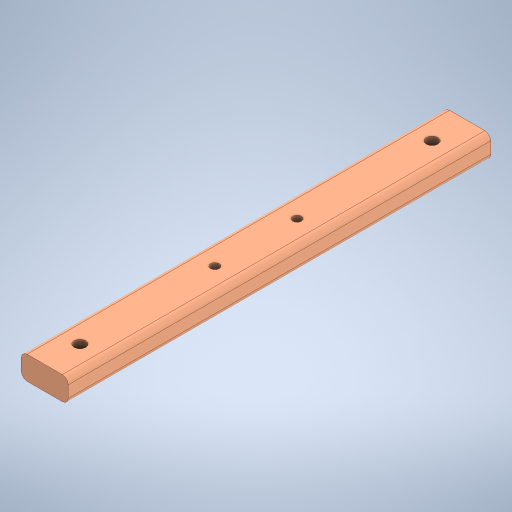
# Autodesk Inventor part: Wood-4
Saved by Autodesk Inventor 2024 (Build 280153000, 153)
## iProperties
Created: 2024-03-20
Part Number: Wood-4
Material: Generic
Document SubType Name: Modeling
Designer: Liz
Density: 1 g/cm^3
Appearance: Default
Author: Liz
Autodesk Inventor part; units mm, degrees
ref_plane "YZ Plane" through (0, 0, 0) normal (1, 0, 0) x (0, 1, 0)
ref_plane "XZ Plane" through (0, 0, 0) normal (0, 1, 0) x (-1, 0, 0)
ref_plane "XY Plane" through (0, 0, 0) normal (0, 0, 1) x (1, 0, 0)
sketch "Sketch1" plane through (0, 0, 0) normal (0, 0, 1) x (1, 0, 0)
  line L0 (-38.1, -25.4) -> (38.1, -25.4)
  line L1 (50.8, -12.7) -> (50.8, 12.7)
  line L2 (38.1, 25.4) -> (-38.1, 25.4)
  line L3 (-50.8, 12.7) -> (-50.8, -12.7)
  line L4 (-50.8, -25.4) -> (50.8, 25.4) construction
  line L5 (50.8, -25.4) -> (-50.8, 25.4) construction
  arc A0 (-38.1, 25.4) -> (-50.8, 12.7) centre (-38.1, 12.7) ccw
  arc A1 (-50.8, -12.7) -> (-38.1, -25.4) centre (-38.1, -12.7) ccw
  arc A2 (38.1, -25.4) -> (50.8, -12.7) centre (38.1, -12.7) ccw
  arc A3 (50.8, 12.7) -> (38.1, 25.4) centre (38.1, 12.7) ccw
  point P0 (0, 0)
  dimension "d0" = 50.8
  dimension "d1" = 101.6
  dimension "d2" = 12.7
  constraints: 12 end point, 8 point on circle, 8 point on line, 8 tangent, 4 centre point, 3 equal radius, 2 midpoint, 2 parallel, 1 horizontal, 1 perpendicular
  measures "d0" distance of L5.end L4.start
  measures "d1" distance of L4.end L5.end
  measures "d2" radius of A0
extrude "Extrusion1" add sketch "Sketch1" along normal blind 914.4
sketch "Sketch2" plane through (-38.1, 25.4, 0) normal (0, 1, 0) x (1, 0, 0)
  circle A0 centre (38.1, -838.2) radius 12.7
  circle A1 centre (38.1, -76.2) radius 12.7
  line L0 (76.2, 0) -> (0, 0) projected
  line L1 (-12.7, 0) -> (-12.7, -914.4) projected
  circle A2 centre (38.1, -546.1) radius 9.525
  circle A3 centre (38.1, -368.3) radius 9.525
  point P0 (38.1, 0)
  point P1 (38.1, 0)
  point P2 (-12.7, -457.2)
  dimension "d5" = 762
  dimension "d6" = 381
  dimension "d7" = 25.4
  dimension "d10" = 177.8
  dimension "d11" = 88.9
  dimension "d12" = 19.05
  constraints: 4 centre point, 4 vertical alignment, 2 equal radius, 2 midpoint
  measures "d5" distance of A1.centre A0.centre
  measures "d6" vertical distance of point (-12.7, -457.2) A0.centre
  measures "d7" diameter of A0
  measures "d10" distance of A3.centre A2.centre
  measures "d11" vertical distance of point (-12.7, -457.2) A2.centre
  measures "d12" diameter of A2
extrude "Extrusion2" cut sketch "Sketch2" against normal blind 609.6
body "Solid1"
